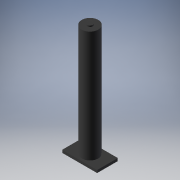
# Autodesk Inventor part: SyringeBody
Saved by Autodesk Inventor 2018 (Build 220112000, 112)
## iProperties
Created: 2017-02-19
Part Number: SyringeBody
Material: Generic
Document SubType Name: Modeling
Designer: Owner
Density: 1 g/cm^3
Appearance: Default
Author: Owner
Autodesk Inventor part; units mm, degrees
ref_plane "YZ Plane" through (0, 0, 0) normal (1, 0, 0) x (0, 1, 0)
ref_plane "XZ Plane" through (0, 0, 0) normal (0, 1, 0) x (-1, 0, 0)
ref_plane "XY Plane" through (0, 0, 0) normal (0, 0, 1) x (1, 0, 0)
sketch "Sketch1" plane through (0, 0, 0) normal (0, 1, 0) x (-1, 0, 0)
  circle A0 centre (0, 0) radius 5.4
  dimension "d0" = 10.8
  constraints: 1 centre point, 1 coincident
  measures "d0" diameter of A0
extrude "Extrusion1" add sketch "Sketch1" along normal blind 73.6
sketch "Sketch2" plane through (0, 0, 0) normal (0, -1, 0) x (1, 0, 0)
  circle A0 centre (0, 0) radius 3.2
  dimension "d3" = 6.4
  constraints: 1 centre point, 1 coincident
  measures "d3" diameter of A0
extrude "Extrusion2" cut sketch "Sketch2" against normal blind 70.8
sketch "Sketch3" plane through (0, 73.6, 0) normal (0, 1, 0) x (1, 0, 0)
  circle A0 centre (0, 0) radius 1.9
  constraints: 1 centre point, 1 coincident
extrude "Extrusion3" add sketch "Sketch3" along normal blind 1
sketch "Sketch4" plane through (0, 0, 0) normal (0, -1, 0) x (1, 0, 0)
  line L0 (0, 0) -> (0, 6.725)
  line L1 (0, 6.725) -> (0, -6.725)
  line L2 (0, 6.725) -> (11.425, 6.725)
  line L3 (11.425, 6.725) -> (-11.425, 6.725)
  line L4 (-11.425, 6.725) -> (-11.425, -2.725)
  line L5 (11.425, -2.725) -> (11.425, 6.725)
  circle A0 centre (0, 0) radius 3.2 projected
  line L6 (-11.425, 6.725) -> (-11.425, -6.725)
  line L7 (-11.425, -6.725) -> (11.425, -6.725)
  line L8 (11.425, -6.725) -> (11.425, 6.725)
  dimension "d8" = 6.725
  dimension "d9" = 13.45
  dimension "d10" = 11.425
  dimension "d11" = 22.85
  dimension "d17" = 13.45
  constraints: 18 end point, 3 perpendicular, 2 horizontal, 2 vertical, 1 point on line
  measures "d8" distance of L0.start L0.end
  measures "d9" distance of L0.end L1.end
  measures "d10" distance of L0.end L2.end
  measures "d11" distance of L2.end L3.end
  measures "d17" distance of L3.end L6.end
extrude "Extrusion4" add sketch "Sketch4" along normal blind 1.75 contours A0 L1 L7 L6 L4 L3 L0 | L0 L2 L5 L8 L7 L1 A0
body "Solid1"
